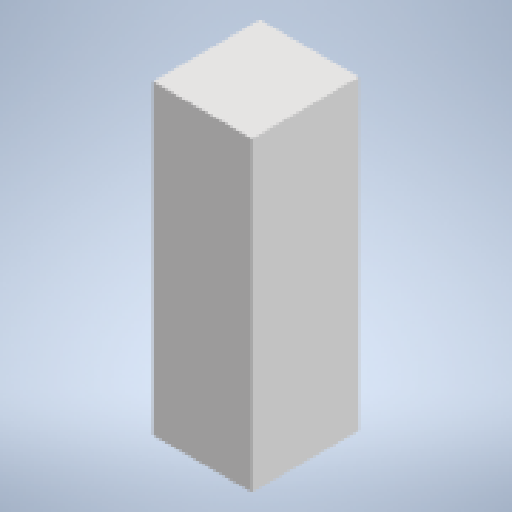
# Autodesk Inventor part: Part5
Saved by Autodesk Inventor 2025.1 (Build 291241020, 241B)
## iProperties
Created: 2025-05-16
Part Number: Part5
Material: Generic
Document SubType Name: Modeling
Designer: tiago
Density: 1 g/cm^3
Appearance: Default
Author: tiago
Autodesk Inventor part; units mm, degrees
ref_plane "YZ Plane" through (0, 0, 0) normal (1, 0, 0) x (0, 1, 0)
ref_plane "XZ Plane" through (0, 0, 0) normal (0, 1, 0) x (-1, 0, 0)
ref_plane "XY Plane" through (0, 0, 0) normal (0, 0, 1) x (1, 0, 0)
sketch "Sketch1" plane through (0, 0, 0) normal (0, 0, 1) x (1, 0, 0)
  line L0 (-4.6348, 14.2907) -> (4.6348, 14.2907)
  line L1 (4.6348, 14.2907) -> (4.6348, -14.2907)
  line L2 (4.6348, -14.2907) -> (-4.6348, -14.2907)
  line L3 (-4.6348, -14.2907) -> (-4.6348, 14.2907)
  line L4 (-4.6348, 14.2907) -> (4.6348, -14.2907) construction
  line L5 (4.6348, 14.2907) -> (-4.6348, -14.2907) construction
  point P0 (0, 0)
  constraints: 12 end point, 2 midpoint, 2 parallel, 1 horizontal, 1 perpendicular
extrude "Extrusion1" add sketch "Sketch1" against normal blind 10
body "Solid1"
